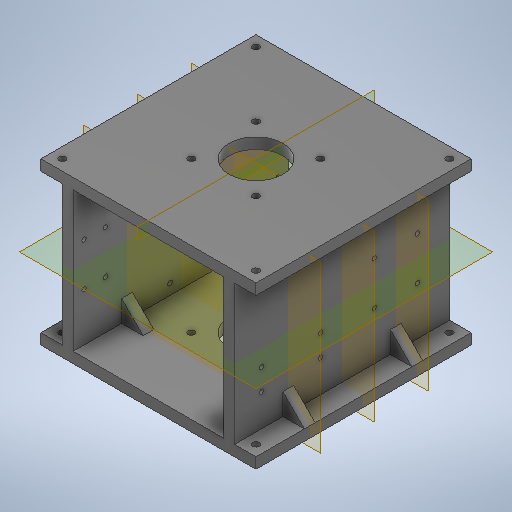
# Autodesk Inventor part: main_case
Saved by Autodesk Inventor 2026.2 (Build 302298010, 298A)
## iProperties
Created: 2026-05-01
Part Number: main_case
Material: ABS Plastic
Document SubType Name: Modeling
Designer: chris
Density: 1.06 g/cm^3
Appearance: Smooth - White
Author: chris
Autodesk Inventor part; units mm, degrees
ref_plane "YZ Plane" through (0, 0, 0) normal (1, 0, 0) x (0, 1, 0)
ref_plane "XZ Plane" through (0, 0, 0) normal (0, 1, 0) x (-1, 0, 0)
ref_plane "XY Plane" through (0, 0, 0) normal (0, 0, 1) x (1, 0, 0)
sketch "Sketch1" plane through (0, 0, 0) normal (0, 1, 0) x (-1, 0, 0)
  line L0 (100, 100) -> (-100, 100)
  line L1 (-100, 100) -> (-100, -100)
  line L2 (-100, -100) -> (100, -100)
  line L3 (100, -100) -> (100, 100)
  line L4 (100, 100) -> (-100, -100) construction
  line L5 (-100, 100) -> (100, -100) construction
  point P0 (0, 0)
  dimension "d0" = 200
  dimension "d1" = 200
  constraints: 12 end point, 2 midpoint, 2 parallel, 1 horizontal, 1 perpendicular
  measures "d0" distance of L2.end L1.end
  measures "d1" distance of L1.end L0.end
extrude "Extrusion1" add sketch "Sketch1" along normal blind 10
sketch "Sketch2" plane through (0, 10, 0) normal (0, 1, 0) x (1, 0, 0)
  line L0 (-80, -100) -> (-70, -100)
  line L1 (-70, -100) -> (-70, 100)
  line L2 (-70, 100) -> (-80, 100)
  line L3 (-80, 100) -> (-80, -100)
  line L4 (-80, -100) -> (-70, 100) construction
  line L5 (-70, -100) -> (-80, 100) construction
  line L6 (80, -100) -> (70, -100)
  line L7 (70, -100) -> (70, 100)
  line L8 (70, 100) -> (80, 100)
  line L9 (80, 100) -> (80, -100)
  line L10 (80, -100) -> (70, 100) construction
  line L11 (70, -100) -> (80, 100) construction
  line L12 (100, 100) -> (-100, 100) projected
  line L13 (-100, -100) -> (100, -100) projected
  line L14 (-100, 100) -> (-100, -100) projected
  line L15 (100, -100) -> (100, 100) projected
  point P0 (0, 0)
  point P1 (-75, 0)
  point P2 (75, 0)
  dimension "d4" = 10
  dimension "d5" = 10
  dimension "d6" = 20
  dimension "d7" = 20
  constraints: 24 end point, 4 collinear, 4 midpoint, 4 parallel, 2 horizontal, 2 perpendicular
  measures "d4" distance of L0.start L0.end
  measures "d5" distance of L6.start L6.end
  measures "d6" distance between parallel lines of L14 L3
  measures "d7" distance between parallel lines of L9 L15
extrude "Extrusion2" add sketch "Sketch2" along normal blind 130 contours L3 L2 L1 L0 | L7 L8 L9 L6
ref_plane "Work Plane1" through (-100, 0, 50) normal (0, 0, 1) x (1, 0, 0)
ref_plane "Work Plane2" through (-100, 0, -50) normal (0, 0, 1) x (1, 0, 0)
sketch "Sketch3" plane through (-100, 0, 50) normal (0, 0, 1) x (1, 0, 0)
  line L0 (180, 10) -> (180, 140) projected
  line L1 (180, 10) -> (200, 10) projected
  line L2 (20, 10) -> (20, 140) projected
  line L3 (0, 10) -> (20, 10) projected
  line L4 (30, 10) -> (30, 140) projected
  line L5 (30, 10) -> (170, 10) projected
  line L6 (170, 10) -> (170, 140) projected
  line L7 (180, 30) -> (200, 10)
  line L8 (170, 30) -> (150, 10)
  line L9 (30, 30) -> (50, 10)
  line L10 (20, 30) -> (0, 10)
  line L11 (20, 30) -> (20, 10)
  line L12 (30, 30) -> (30, 10)
  line L13 (170, 30) -> (170, 10)
  line L14 (180, 30) -> (180, 10)
  point P0 (100, 0)
  dimension "d12" = 20
  dimension "d13" = 20
  dimension "d14" = 20
  dimension "d15" = 20
  dimension "d16" = 20
  dimension "d17" = 20
  dimension "d19" = 20
  constraints: 16 end point, 8 point on line, 2 perpendicular, 1 collinear, 1 vertical
  measures "d12" distance from line of L1 L7.start
  measures "d13" distance from line of L0 L7.end
  measures "d14" distance from line of L6 L8.end
  measures "d15" distance from line of L5 L8.start
  measures "d16" distance from line of L5 L9.start
  measures "d17" distance from line of L4 L9.end
  measures "d19" distance from line of L3 L10.start
extrude "Extrusion3" add sketch "Sketch3" along normal mid plane 10
ref_plane "Work Plane3" through (-100, 0, 0) normal (0, 0, 1) x (1, 0, 0)
mirror "Mirror1" about plane through (-100, 0, 0) normal (0, 0, 1) of "Extrusion3"
ref_plane "Work Plane4" through (0, 75, 0) normal (0, -1, 0) x (1, 0, 0)
sketch "Sketch4" plane through (0, 140, 0) normal (0, 1, 0) x (1, 0, 0)
  line L0 (-100, -100) -> (100, -100)
  line L1 (100, -100) -> (100, 100)
  line L2 (100, 100) -> (-100, 100)
  line L3 (-100, 100) -> (-100, -100)
  line L4 (-100, -100) -> (100, 100) construction
  line L5 (100, -100) -> (-100, 100) construction
  point P0 (0, 0)
  dimension "d24" = 200
  dimension "d25" = 200
  constraints: 12 end point, 2 midpoint, 2 parallel, 1 horizontal, 1 perpendicular
  measures "d24" distance of L2.end L1.end
  measures "d25" distance of L1.end L0.end
extrude "Extrusion4" add sketch "Sketch4" along normal blind 10
mirror "Mirror2" about plane through (0, 75, 0) normal (0, -1, 0) of "Extrusion3", "Mirror1"
sketch "Sketch5" plane through (0, 0, 0) normal (0, -1, 0) x (1, 0, 0)
  circle A0 centre (0, 0) radius 25
  dimension "d28" = 50
  constraints: 1 centre point, 1 coincident
  measures "d28" diameter of A0
extrude "Extrusion5" cut sketch "Sketch5" against normal through all
sketch "Sketch6" plane through (0, 0, 0) normal (0, -1, 0) x (1, 0, 0)
  circle A0 centre (-90, -90) radius 3.1
  line L0 (100, -100) -> (-100, -100) projected
  line L1 (-100, -100) -> (-100, 100) projected
  point P0 (0, 0)
  dimension "d31" = 6.2
  dimension "d32" = 10
  dimension "d33" = 10
  constraints: 1 centre point
  measures "d31" diameter of A0
  measures "d32" distance from line of L0 A0.centre
  measures "d33" distance from line of L1 A0.centre
extrude "Extrusion6" cut sketch "Sketch6" against normal through all
ref_plane "Work Plane5" through (0, 140, 100) normal (-1, 0, 0) x (0, 0, 1)
mirror "Mirror3" about plane through (-100, 0, 0) normal (0, 0, 1) of "Extrusion6"
mirror "Mirror4" about plane through (0, 140, 100) normal (-1, 0, 0) of "Extrusion6", "Mirror3"
sketch "Sketch8" plane through (0, 150, 0) normal (0, 1, 0) x (1, 0, 0)
  circle A0 centre (-30, -30) radius 3.1
  line L0 (140, 0) -> (-140, 0) projected
  line L1 (0, -140) -> (0, 140) projected
  point P0 (0, 0)
  dimension "d37" = 6.2
  dimension "d38" = 30
  dimension "d39" = 30
  constraints: 1 centre point
  measures "d37" diameter of A0
  measures "d38" distance from line of L0 A0.centre
  measures "d39" distance from line of A0.centre L1
extrude "Extrusion7" cut sketch "Sketch8" against normal through all
mirror "Mirror5" about plane through (-100, 0, 0) normal (0, 0, 1) of "Extrusion7"
mirror "Mirror6" about plane through (0, 140, 100) normal (-1, 0, 0) of "Extrusion7", "Mirror5"
sketch "Sketch9" plane through (-80, 10, 55) normal (-1, 0, 0) x (0, 0, 1)
  circle A0 centre (-45, 10) radius 2.05
  circle A1 centre (-45, 62) radius 2.05
  circle A2 centre (-82, 10) radius 2.05
  circle A3 centre (-88, 62) radius 2.05
  line L0 (-10, 0) -> (-100, 0) projected
  line L1 (45, 0) -> (45, 130) projected
  point P0 (-55, -10)
  dimension "d42" = 4.1
  dimension "d43" = 4.1
  dimension "d44" = 52
  dimension "d45" = 0
  dimension "d46" = 4.1
  dimension "d47" = 37
  dimension "d48" = 4.1
  dimension "d49" = 43
  dimension "d50" = 10
  dimension "d51" = 0
  dimension "d52" = 0
  dimension "d53" = 90
  constraints: 4 centre point
  measures "d42" diameter of A0
  measures "d43" diameter of A1
  measures "d44" distance of A1.centre A0.centre
  measures "d45" horizontal distance of A0.centre A1.centre
  measures "d46" diameter of A2
  measures "d47" distance of A0.centre A2.centre
  measures "d48" diameter of A3
  measures "d49" distance of A3.centre A1.centre
  measures "d50" distance from line of L0 A0.centre
  measures "d51" vertical distance of A0.centre A2.centre
  measures "d52" vertical distance of A3.centre A1.centre
  measures "d53" distance from line of L1 A0.centre
hole "Hole1" at (-80, 72, -33) at (-80, 72, 10) at (-80, 20, 10) at (-80, 20, -27) direction (1, 0, 0) diameter 4.5 depth 10 tip angle 118
sketch "Sketch10" plane through (80, 10, 100) normal (1, 0, 0) x (0, 0, -1)
  circle A0 centre (80, 30) radius 2.05
  circle A1 centre (25, 30) radius 2.05
  circle A2 centre (25, 50) radius 2.05
  circle A3 centre (80, 50) radius 2.05
  line L0 (145, 0) -> (55, 0) projected
  line L1 (200, 0) -> (200, 130) projected
  point P0 (100, -10)
  dimension "d61" = 4.1
  dimension "d62" = 4.1
  dimension "d63" = 4.1
  dimension "d64" = 4.1
  dimension "d65" = 0
  dimension "d66" = 55
  dimension "d67" = 0
  dimension "d68" = 20
  dimension "d69" = 0
  dimension "d70" = 0
  dimension "d71" = 30
  dimension "d74" = 120
  constraints: 4 centre point
  measures "d61" diameter of A0
  measures "d62" diameter of A1
  measures "d63" diameter of A2
  measures "d64" diameter of A3
  measures "d65" vertical distance of A1.centre A0.centre
  measures "d66" distance of A0.centre A1.centre
  measures "d67" horizontal distance of A0.centre A3.centre
  measures "d68" distance of A0.centre A3.centre
  measures "d69" vertical distance of A3.centre A2.centre
  measures "d70" horizontal distance of A1.centre A2.centre
  measures "d71" distance from line of L0 A0.centre
  measures "d74" distance from line of L1 A0.centre
extrude "Extrusion8" cut sketch "Sketch10" against normal blind 10
sketch "Sketch11" plane through (80, 10, 100) normal (1, 0, 0) x (0, 0, -1)
  circle A0 centre (170, 85) radius 2.05
  circle A1 centre (170, 45) radius 2.05
  circle A2 centre (130, 45) radius 2.05
  circle A3 centre (130, 85) radius 2.05
  line L0 (150, -40) -> (150, 170) projected
  line L1 (240, 65) -> (-40, 65) projected
  point P0 (100, -10)
  dimension "d75" = 4.1
  dimension "d76" = 4.1
  dimension "d77" = 4.1
  dimension "d78" = 4.1
  dimension "d79" = 20
  dimension "d80" = 20
  dimension "d81" = 20
  dimension "d82" = 20
  dimension "d83" = 20
  dimension "d84" = 20
  dimension "d85" = 20
  dimension "d86" = 20
  constraints: 4 centre point
  measures "d75" diameter of A0
  measures "d76" diameter of A1
  measures "d77" diameter of A2
  measures "d78" diameter of A3
  measures "d79" distance from line of A0.centre L0
  measures "d80" distance from line of L1 A0.centre
  measures "d81" distance from line of L1 A1.centre
  measures "d82" distance from line of L0 A1.centre
  measures "d83" distance from line of L0 A2.centre
  measures "d84" distance from line of L1 A2.centre
  measures "d85" distance from line of L1 A3.centre
  measures "d86" distance from line of L0 A3.centre
extrude "Extrusion9" cut sketch "Sketch11" against normal blind 10
sketch "Sketch12" plane through (-80, 10, 55) normal (-1, 0, 0) x (0, 0, 1)
  circle A0 centre (15, 85) radius 2.05
  circle A1 centre (15, 45) radius 2.05
  line L0 (85, 65) -> (-195, 65) projected
  line L1 (-5, 170) -> (-5, -40) projected
  circle A2 centre (35, 85) radius 2.05
  circle A3 centre (35, 45) radius 2.05
  point P0 (-55, -10)
  dimension "d89" = 4.1
  dimension "d90" = 4.1
  dimension "d91" = 20
  dimension "d92" = 20
  dimension "d93" = 20
  dimension "d94" = 20
  dimension "d95" = 4.1
  dimension "d96" = 4.1
  dimension "d97" = 40
  dimension "d98" = 40
  dimension "d99" = 20
  dimension "d100" = 20
  constraints: 4 centre point
  measures "d89" diameter of A0
  measures "d90" diameter of A1
  measures "d91" distance from line of L0 A0.centre
  measures "d92" distance from line of L1 A0.centre
  measures "d93" distance from line of L1 A1.centre
  measures "d94" distance from line of L0 A1.centre
  measures "d95" diameter of A2
  measures "d96" diameter of A3
  measures "d97" distance from line of L1 A3.centre
  measures "d98" distance from line of L1 A2.centre
  measures "d99" distance from line of L0 A2.centre
  measures "d100" distance from line of L0 A3.centre
extrude "Extrusion10" cut sketch "Sketch12" against normal blind 10
mirror "Mirror7" about plane through (-100, 0, 0) normal (0, 0, 1) of "Extrusion10"
body "Solid1"
